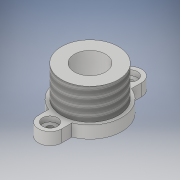
# Autodesk Inventor part: prensa_cabo_fixador
Saved by Autodesk Inventor 2019.4 (Build 234330000, 330)
## iProperties
Created: 2021-02-09
Part Number: prensa_cabo_fixador
Material: Genérico
Document SubType Name: Modeling
Designer: Lattes
Density: 1 g/cm^3
Appearance: Padrão
Author: Lattes
Autodesk Inventor part; units mm, degrees
ref_plane "YZ Plane" through (0, 0, 0) normal (1, 0, 0) x (0, 1, 0)
ref_plane "XZ Plane" through (0, 0, 0) normal (0, 1, 0) x (-1, 0, 0)
ref_plane "XY Plane" through (0, 0, 0) normal (0, 0, 1) x (1, 0, 0)
sketch "Esboço1" plane through (0, 0, 0) normal (0, 1, 0) x (-1, 0, 0)
  circle A0 centre (0, 0) radius 12.3
  dimension "d0" = 24.6
  constraints: 1 centre point, 1 coincident
  measures "d0" diameter of A0
extrude "Extrusão1" add sketch "Esboço1" along normal blind 4.75
sketch "Esboço2" plane through (0, 0, 0) normal (0, -1, 0) x (1, 0, 0)
  circle A0 centre (0, 0) radius 7.775
  dimension "d3" = 15.55
  constraints: 1 centre point, 1 coincident
  measures "d3" diameter of A0
extrude "Extrusão2" add sketch "Esboço2" along normal blind 1.25
sketch "Esboço3" plane through (0, 0, 0) normal (0, -1, 0) x (1, 0, 0)
  circle A0 centre (0, 0) radius 12.3 projected
  circle A1 centre (0, -15.425) radius 1.25
  line L0 (-4.5, -15.425) -> (-4.5, -11.4473)
  line L1 (4.5, -15.425) -> (4.5, -11.4473)
  line L2 (4.5, -15.425) -> (8.4777, -15.425) construction
  arc A2 (-4.5, -15.425) -> (4.5, -15.425) centre (0, -15.425) ccw
  dimension "d12" = 90
  constraints: 6 end point, 4 point on circle, 2 centre point, 1 horizontal, 1 perpendicular
  measures "d12" angle of L2 L1
extrude "Extrusão3" add sketch "Esboço3" against normal blind 4.75 contours A0 L1 A2 L0
sketch "Esboço4" plane through (0, 4.75, 0) normal (0, 1, 0) x (1, 0, 0)
  circle A0 centre (0, 15.425) radius 1.25 projected
  circle A1 centre (0, 15.425) radius 2.9
  point P0 (0, 0)
  dimension "d15" = 5.8
  constraints: 1 centre point, 1 coincident
  measures "d15" diameter of A1
extrude "Extrusão4" cut sketch "Esboço4" against normal blind 2
pattern_circular "Padrão circular1" count 2 over 360 about axis through (0, 0, 0) along (0, 1, 0) of "Extrusão3", "Extrusão4"
sketch "Esboço5" plane through (0, 4.75, 0) normal (0, 1, 0) x (1, 0, 0)
  circle A0 centre (0, 0) radius 11
  dimension "d21" = 22
  constraints: 1 centre point, 1 coincident
  measures "d21" diameter of A0
extrude "Extrusão5" add sketch "Esboço5" along normal blind 12
sketch "Esboço6" plane through (0, 16.75, 0) normal (0, 1, 0) x (1, 0, 0)
  circle A0 centre (0, 0) radius 6
  dimension "d24" = 12
  constraints: 1 centre point, 1 coincident
  measures "d24" diameter of A0
extrude "Extrusão6" cut sketch "Esboço6" against normal blind 20
thread "Rosca1" size "M22x3" class "6g" standard "ANSI Metric M Profile" full length
sketch "Esboço7" plane through (0, 0, 0) normal (0, -1, 0) x (1, 0, 0)
  circle A0 centre (0, -15.425) radius 1.25 projected
  circle A1 centre (0, -15.425) radius 1.5
  circle A2 centre (0, 15.425) radius 1.25 projected
  circle A3 centre (0, 15.425) radius 1.5
  circle A4 centre (0, 0) radius 8
  line L0 (-14, 21.425) -> (14, 21.425)
  line L1 (14, 21.425) -> (14, -21.425)
  line L2 (14, -21.425) -> (-14, -21.425)
  line L3 (-14, -21.425) -> (-14, 21.425)
  dimension "d29" = 3
  dimension "d30" = 3
  dimension "d31" = 16
  constraints: 8 end point, 3 centre point, 3 coincident, 2 parallel, 1 horizontal, 1 perpendicular
  measures "d29" diameter of A1
  measures "d30" diameter of A3
  measures "d31" diameter of A4
